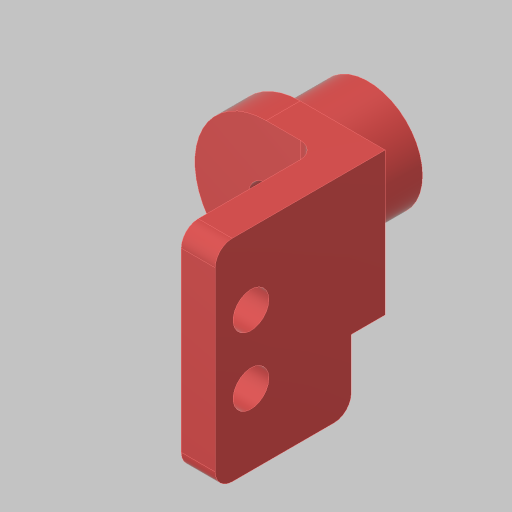
# Autodesk Inventor part: EL2-020
Saved by Autodesk Inventor 2023.5 (Build 275446000, 446)
## iProperties
Created: 2025-01-21
Part Number: EL2-020
Material: ABS Plastic
Document SubType Name: Modeling
Designer: slick
Density: 1.06 g/cm^3
Appearance: Smooth - Red
Author: slick
Autodesk Inventor part; units mm, degrees
ref_plane "YZ Plane" through (0, 0, 0) normal (1, 0, 0) x (0, 1, 0)
ref_plane "XZ Plane" through (0, 0, 0) normal (0, 1, 0) x (-1, 0, 0)
ref_plane "XY Plane" through (0, 0, 0) normal (0, 0, 1) x (1, 0, 0)
sketch "Sketch1" plane through (0, 0, 0) normal (0, 0, 1) x (1, 0, 0)
  circle A0 centre (0, 0) radius 10.16
  circle A1 centre (0, 0) radius 8.7376
  dimension "d0" = 20.32
  dimension "d6" = 17.4752
  constraints: 2 centre point, 2 coincident
  measures "d0" diameter of A0
  measures "d6" diameter of A1
extrude "Extrusion1" add sketch "Sketch1" along normal blind 12.7 contours A0 | A1
sketch "Sketch2" plane through (0, 0, 12.7) normal (0, 0, 1) x (1, 0, 0)
  circle A0 centre (0, 0) radius 10.16 projected
  circle A1 centre (0, 0) radius 13.335 construction
  line L0 (0, 13.335) -> (15.875, 13.335)
  line L1 (15.875, 13.335) -> (15.875, -13.335)
  line L2 (15.875, -13.335) -> (0, -13.335)
  arc A2 (0, 13.335) -> (0, -13.335) centre (0, 0) ccw
  point P0 (15.875, 0)
  dimension "d3" = 3.175
  dimension "d14" = 15.875
  constraints: 6 end point, 4 point on circle, 2 centre point, 2 horizontal, 1 coincident, 1 horizontal alignment, 1 midpoint, 1 perpendicular, 1 tangent
  measures "d3" radial gap between concentric circles of A0 A1
  measures "d14" distance of L0.start L0.end
extrude "Extrusion2" add sketch "Sketch2" along normal blind 6.35 contours A0 | L0 L1 L2 A2
sketch "Sketch4" plane through (0, 0, 19.05) normal (0, 0, 1) x (1, 0, 0)
  arc A0 (0, 13.335) -> (0, -13.335) centre (0, 0) ccw projected
  constraints: 1 coincident
hole "Hole2" at (0, 0, 19.05) direction (0, 0, -1) diameter 6.5278 end through all clearance for "Flat Head Machine Screw (82)" size "1/4" standard "Ansi Unified Screw Threads"
sketch "Sketch5" plane through (0, 0, 19.05) normal (0, 0, 1) x (1, 0, 0)
  line L0 (15.875, 13.335) -> (0, 13.335) projected
  line L1 (0, -13.335) -> (15.875, -13.335) projected
  line L2 (15.875, 13.335) -> (9.525, 13.335)
  line L3 (9.525, 13.335) -> (9.525, -13.335)
  line L4 (9.525, -13.335) -> (15.875, -13.335)
  line L5 (15.875, -13.335) -> (15.875, 13.335)
  line L6 (9.525, -13.335) -> (15.875, -13.335)
  line L7 (15.875, -13.335) -> (15.875, -26.035)
  line L8 (15.875, -26.035) -> (9.525, -26.035)
  line L9 (9.525, -26.035) -> (9.525, -13.335)
  point P0 (0, 0)
  point P1 (15.875, -19.685)
  point P2 (15.875, 0)
  dimension "d22" = 6.35
  dimension "d36" = 12.7
  constraints: 16 end point, 4 parallel, 2 horizontal, 2 midpoint, 2 perpendicular, 1 point on line, 1 vertical alignment
  measures "d22" distance between parallel lines of L5 L3
  measures "d36" distance between parallel lines of L1 L8
extrude "Extrusion3" add sketch "Sketch5" along normal blind 25.4
fillet "Fillet1" radius 3.175 4 edges at (9.525, 0, 19.05) (12.7, -26.035, 19.05) (12.7, -26.035, 44.45) (12.7, 13.335, 44.45)
sketch "Sketch6" plane through (15.875, -13.335, 12.7) normal (1, 0, 0) x (0, 0, -1)
  line L0 (-25.0698, 13.335) -> (-25.0698, 0.635) construction
  line L1 (0, 26.67) -> (-28.575, 26.67) construction
  line L2 (-31.75, -9.525) -> (-31.75, 23.495) projected
  point P0 (12.7, 13.335)
  point P1 (-25.0698, 6.985)
  dimension "d26" = 12.7
  dimension "d35" = 13.335
  dimension "d37" = 6.6802
  constraints: 2 end point, 1 midpoint, 1 vertical, 1 vertical alignment
  measures "d26" distance of L0.start L0.end
  measures "d35" distance from line of L1 L0.start
  measures "d37" distance between parallel lines of L0 L2
hole "Hole3" at (15.875, 0, 37.7698) at (15.875, -12.7, 37.7698) direction (-1, 0, 0) diameter 6.7 end through all
body "Solid1"
